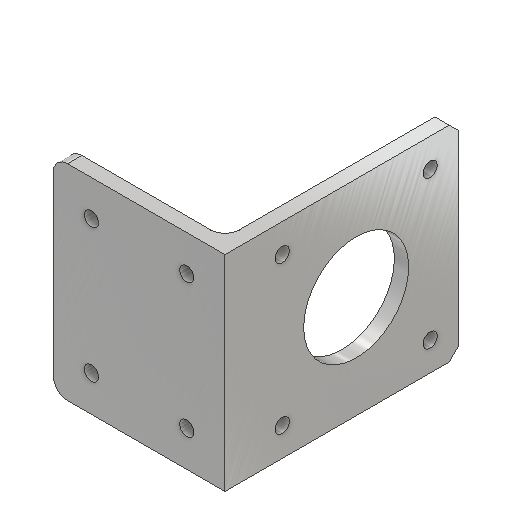
# Autodesk Inventor part: CNCM_ALU_X_Axis_Nema_17_Mount
Saved by Autodesk Inventor 2026.1 (Build 301233000, 233)
## iProperties
Created: 2016-03-27
Part Number: CNCM_ALU_X_Axis_Nema_17_Mount
Material: Ogólny
Document SubType Name: Modeling
Designer: Andrzej
Density: 1 g/cm^3
Appearance: Obrobione - aluminium
Mass: 9.32709 g
Surface Area: 72.8124 cm^2
Volume: 9.32709 cm^3
Author: Andrzej
Autodesk Inventor part; units mm, degrees
ref_plane "YZ Plane" through (0, 0, 0) normal (1, 0, 0) x (0, 1, 0)
ref_plane "XZ Plane" through (0, 0, 0) normal (0, 1, 0) x (-1, 0, 0)
ref_plane "XY Plane" through (0, 0, 0) normal (0, 0, 1) x (1, 0, 0)
sketch "Szkic1" plane through (0, 0, 0) normal (0, 0, 1) x (1, 0, 0)
  line L0 (-15.1556, -3.6171) -> (-15.1556, -6.6171)
  line L1 (-15.1556, -6.6171) -> (20.8444, -6.6171)
  line L2 (20.8444, -6.6171) -> (20.8444, 42.3829)
  line L3 (20.8444, 42.3829) -> (17.8444, 42.3829)
  line L4 (17.8444, 42.3829) -> (17.8444, -3.6171)
  line L5 (17.8444, -3.6171) -> (-15.1556, -3.6171)
  point P0 (0, 0)
  dimension "d0" = 3
  dimension "d1" = 36
  dimension "d2" = 49
  dimension "d3" = 3
  constraints: 12 end point, 5 perpendicular, 1 vertical
  measures "d0" distance of L0.start L0.end
  measures "d1" distance of L0.end L1.end
  measures "d2" distance of L1.end L2.end
  measures "d3" distance of L2.end L3.end
extrude "Wyciągnięcie proste1" add sketch "Szkic1" along normal blind 43
fillet "Zaokrąglenie1" radius 3 1 edges at (17.8444, -3.6171, 21.5)
sketch "Szkic2" plane through (17.8444, 42.3829, 0) normal (-1, 0, 0) x (0, 0, 1)
  circle A0 centre (21.5033, -21.5) radius 11
  circle A1 centre (21.5, -21.5) radius 16.25
  line L0 (0, 0) -> (0, -43) projected
  line L1 (0, 0) -> (43, 0) projected
  line L2 (43, 0) -> (43, -43) projected
  line L3 (0.5, -0.5) -> (42.5, -0.5)
  line L4 (42.5, -0.5) -> (42.5, -42.5)
  line L5 (42.5, -42.5) -> (0.5, -42.5)
  line L6 (0.5, -42.5) -> (0.5, -0.5)
  point P0 (0, -42.3829)
  point P1 (37, -37)
  point P2 (37, -6)
  point P3 (6, -6)
  point P4 (6, -37)
  dimension "d61" = 42
  dimension "d62" = 42
  dimension "d63" = 0.5
  dimension "d64" = 0.5
  dimension "d65" = 5.5
  dimension "d66" = 5.5
  dimension "d67" = 5.5
  dimension "d68" = 5.5
  dimension "d69" = 5.5
  dimension "d70" = 5.5
  dimension "d71" = 5.5
  dimension "d72" = 5.5
  dimension "d73" = 21
  dimension "d74" = 21
  constraints: 8 end point, 2 centre point, 2 parallel, 1 horizontal, 1 perpendicular
  measures "d61" distance of L4.end L5.end
  measures "d62" distance of L3.end L4.end
  measures "d63" distance between parallel lines of L0 L6
  measures "d64" distance between parallel lines of L1 L3
  measures "d65" distance from line of L6 point (6, -6)
  measures "d66" distance from line of L3 point (6, -6)
  measures "d67" distance from line of L3 point (37, -6)
  measures "d68" distance from line of L4 point (37, -6)
  measures "d69" distance from line of L4 point (37, -37)
  measures "d70" distance from line of L5 point (37, -37)
  measures "d71" distance from line of L5 point (6, -37)
  measures "d72" distance from line of L6 point (6, -37)
  measures "d73" distance from line of A1.centre L6
  measures "d74" distance from line of L3 A0.centre
extrude "Wyciągnięcie proste2" cut sketch "Szkic2" against normal blind 43 contours A0
hole "Otwór1" at (17.8444, 5.3829, 6) at (17.8444, 36.3829, 6) at (17.8444, 36.3829, 37) at (17.8444, 5.3829, 37) direction (1, 0, 0) diameter 3 end through all
chamfer "Faza1" distance 2 angle 45 2 edges at (19.3444, 42.3829, 43) (19.3444, 42.3829, 0)
fillet "Zaokrąglenie2" radius 3 2 edges at (-15.1556, -5.1171, 0) (-15.1556, -5.1171, 43)
sketch "Szkic3" plane through (20.8444, -6.6171, 0) normal (0, -1, 0) x (1, 0, 0)
  arc A0 (-33, 43) -> (-36, 40) centre (-33, 40) ccw projected
  line L0 (-36, 3) -> (-36, 40) projected
  arc A1 (-36, 3) -> (-33, 0) centre (-33, 3) ccw projected
  line L1 (-33, 0) -> (0, 0) projected
  line L2 (0, 0) -> (0, 43) projected
  line L3 (-33, 43) -> (0, 43) projected
  point P0 (-20.8444, 0)
  point P1 (-28, 7.5)
  point P2 (-8, 7.5)
  point P3 (-28, 35.5)
  point P4 (-8, 35.5)
  dimension "d32" = 20
  dimension "d33" = 20
  dimension "d34" = 36
  dimension "d35" = 8
  dimension "d36" = 8
  dimension "d37" = 7.5
  dimension "d38" = 7.5
  dimension "d39" = 7.5
  dimension "d40" = 7.5
  measures "d32" distance of point (-28, 7.5) point (-8, 7.5)
  measures "d33" distance of point (-8, 35.5) point (-28, 35.5)
  measures "d34" distance between parallel lines of L2 L0
  measures "d35" distance from line of L0 point (-28, 7.5)
  measures "d36" distance from line of L0 point (-28, 35.5)
  measures "d37" distance from line of L1 point (-28, 7.5)
  measures "d38" distance from line of L1 point (-8, 7.5)
  measures "d39" distance from line of L3 point (-28, 35.5)
  measures "d40" distance from line of L3 point (-8, 35.5)
hole "Otwór2" at (-7.1556, -6.6171, 7.5) at (12.8444, -6.6171, 7.5) at (-7.1556, -6.6171, 35.5) at (12.8444, -6.6171, 35.5) direction (0, 1, 0) diameter 3 end through all
sketch "Szkic4" plane through (14.8444, -3.6171, 43) normal (0, 1, 0) x (1, 0, 0)
  circle A0 centre (-2, 7.5) radius 1.5 projected
  circle A1 centre (-2, 35.5) radius 1.5 projected
  circle A2 centre (-2, 7.5) radius 3.1
  circle A3 centre (-2, 35.5) radius 3.1
  point P0 (-14.8444, 43)
  dimension "d48" = 6.2
  dimension "d49" = 6.2
  constraints: 2 centre point, 2 coincident
  measures "d48" diameter of A2
  measures "d49" diameter of A3
extrude "Wyciągnięcie proste3" cut sketch "Szkic4" along normal blind 2
equation "\"d66\" = d65"
equation "\"d67\" = d65"
equation "\"d68\" = d65"
equation "\"d69\" = d65"
equation "\"d70\" = d65"
equation "\"d71\" = d65"
equation "\"d72\" = d65"
equation "\"d35\" = -0.5 * d32 + 0.5 * d34"
equation "\"d36\" = d35"
equation "\"d38\" = d37"
equation "\"d39\" = d37"
equation "\"d40\" = d37"
